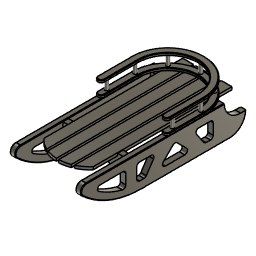
P9 (Autodesk Fusion 360 design; units mm, degrees)
Autodesk Fusion 360 part; units mm, degrees
ref_plane "WorkPlane1" through (300, 0, 0) normal (1, 0, 0) x (0, 1, 0)
sketch "Sketch1" plane through (300, 0, 0) normal (1, 0, 0) x (0, 1, 0)
  arc A0 (-924.4998, 0) -> (-300, -300) centre (-300, 500) ccw
  line L0 (-300, -300) -> (500, -300)
  line L1 (0, 0) -> (0, -300) construction
  line L2 (-924.4998, 0) -> (0, 0)
  line L3 (450, 0) -> (0, 0)
  arc A1 (500, -300) -> (650, -150) centre (500, -150) ccw
  line L4 (650, -150) -> (600, -150)
  arc A2 (450, 0) -> (600, -150) centre (600, 0) ccw
  point P0 (600, 0)
  point P1 (600, 0)
  dimension "d3" = 500
  dimension "d4" = 800
  dimension "d6" = 450
  dimension "d7" = 800
  dimension "d8" = 150
  dimension "d9" = 300
  constraint horizontal L0
  constraint tangent A0 L0
  constraint coincident L0 L1.end
  constraint vertical L1
  constraint coincident L1.start L2.end
  constraint horizontal L2
  constraint horizontal L3
  constraint tangent L0 A1
  constraint horizontal L4
  constraint tangent L4 A2
  constraint equal A1 A2
  constraint coincident P1 P0
  constraint horizontal L1.start P1
  measures "d3" distance of L0.end L1.end
  measures "d4" radius of A0
  measures "d6" distance of L3.start L1.start
  measures "d7" distance of A0.end L0.end
  measures "d8" radius of A1
  measures "d9" distance of L0 L3
extrude "Extrude1" add sketch "Sketch1" along normal mid plane 50 makes body 1
fillet "Fillet1" radius 50 1 edges at (300, -924.4998, 0) on bodies 1
mirror "Mirror1" about plane through (0, 0, 0) normal (1, 0, 0) of bodies 1 makes body 2
sketch "Sketch2" plane through (325, 0, 0) normal (1, 0, 0) x (0, 1, 0)
  arc A0 (-809.902, 0) -> (-843.8954, -86.6667) centre (-809.902, -50) ccw
  arc A1 (-843.8954, -86.6667) -> (-300, -300) centre (-300, 500) ccw
  line L0 (-300, -300) -> (500, -300)
  arc A2 (500, -300) -> (650, -150) centre (500, -150) ccw
  line L1 (650, -150) -> (600, -150)
  arc A3 (450, 0) -> (600, -150) centre (600, 0) ccw
  line L2 (450, 0) -> (-809.902, 0)
  line L3 (0, 0) -> (0, -300) construction
  line L4 (150, -225) -> (-150, -225)
  line L5 (-350, -75) -> (-350, -225)
  line L6 (-350, -225) -> (-270, -225)
  line L7 (-270, -225) -> (-170, -75)
  line L8 (-170, -75) -> (-350, -75)
  line L9 (270, -225) -> (170, -75)
  line L10 (170, -75) -> (350, -75)
  line L11 (350, -75) -> (350, -225)
  line L12 (350, -225) -> (270, -225)
  line L13 (-450, -75) -> (-760, -75)
  line L14 (-450, -75) -> (-450, -225)
  arc A4 (-760, -75) -> (-450, -225) centre (-291.5323, 497.8333) ccw
  line L15 (-150, -225) -> (0, -75)
  line L16 (150, -225) -> (0, -75)
  dimension "d17" = 300
  dimension "d18" = 75
  dimension "d19" = 80
  dimension "d20" = 180
  dimension "d23" = 350
  dimension "d24" = 740
  dimension "d25" = 75
  dimension "d26" = 310
  dimension "d27" = 450
  dimension "d28" = 75
  constraint coincident L3.start origin
  constraint coincident L0 L3.end
  constraint vertical L3
  constraint horizontal L8
  constraint collinear L4 L6
  constraint symmetric L3 L5.start L10.end
  constraint symmetric L3 L5.end L11.end
  constraint symmetric L3 L6.end L9.start
  constraint symmetric L3 L7.end L9.end
  constraint horizontal L13
  constraint perpendicular L13 L14
  constraint equal L5 L14
  constraint collinear L8 L13
  constraint coincident L3 L15.end
  constraint perpendicular L15 L16
  measures "d17" distance of L4.start L4.end
  measures "d18" distance of L0 L4
  measures "d19" distance of L5.end L6.end
  measures "d20" distance of L5.start L7.end
  measures "d23" distance of L3 L5
  measures "d24" radius of A4
  measures "d25" distance of L2 L13
  measures "d26" distance of L13.end L14
  measures "d27" distance of L3 L14
  measures "d28" distance of L2 L15.end
extrude "Extrude2" cut sketch "Sketch2" against normal blind 650 contours L4 L15 L16 | L5 L6 L7 L8 | L9 L10 L11 L12 | L13 L14 A4 bodies 1 2
fillet "Fillet2" radius 25 28 edges at (300, -450, -75) (300, -450, -225) (300, -760, -75) (300, -350, -225) (300, -270, -225) (300, -350, -75) (300, -170, -75) (300, 0, -75) (300, 150, -225) (300, -150, -225) (300, 170, -75) (300, 270, -225) (300, 350, -225) (300, 350, -75) (-300, 350, -75) (-300, 0, -75) (-300, 350, -225) (-300, 150, -225) (-300, 270, -225) (-300, -150, -225) (-300, 170, -75) (-300, -350, -75) (-300, -760, -75) (-300, -170, -75) (-300, -270, -225) (-300, -450, -225) (-300, -450, -75) (-300, -350, -225) on bodies 1 2
fillet "Fillet3" radius 5 20 edges at (325, -179.951, 0) (325, -856.4494, -31.7426) (325, -592.1187, -244.7595) (325, 100, -300) (325, 606.066, -256.066) (275, 606.066, -256.066) (275, 100, -300) (275, -592.1187, -244.7595) (275, -856.4494, -31.7426) (275, -179.951, 0) (-275, 606.066, -256.066) (-275, 100, -300) (-275, -592.1187, -244.7595) (-275, -856.4494, -31.7426) (-275, -179.951, 0) (-325, -179.951, 0) (-325, -856.4494, -31.7426) (-325, -592.1187, -244.7595) (-325, 100, -300) (-325, 606.066, -256.066) on bodies 1 2
ref_plane "WorkPlane2" through (0, -425, 0) normal (0, 1, 0) x (0, 0, 1)
sketch "Sketch3" plane through (0, -425, 0) normal (0, 1, 0) x (1, 0, 0)
  line L0 (-275, 5) -> (-225, 5)
  line L1 (-225, 5) -> (-225, 25)
  line L2 (-225, 25) -> (-2.6918, 25)
  line L3 (-275, 5) -> (-275, 155)
  line L4 (-275, 155) -> (-198.4313, 155)
  line L5 (0, 0) -> (0, 80) construction
  arc A0 (-198.4313, 155) -> (0, 80) centre (0, 380) ccw
  line L6 (225, 25) -> (2.6918, 25)
  line L7 (225, 5) -> (225, 25)
  line L8 (275, 5) -> (225, 5)
  line L9 (275, 5) -> (275, 155)
  line L10 (275, 155) -> (198.4313, 155)
  arc A1 (0, 80) -> (198.4313, 155) centre (0, 380) ccw
  line L11 (-2.6918, 25) -> (0, 25)
  line L12 (0, 25) -> (2.6918, 25)
  point P0 (-275, 5)
  point P1 (-275, 5)
  point P2 (-325, 5)
  dimension "d36" = 150
  dimension "d37" = 5
  dimension "d38" = 50
  dimension "d39" = 20
  dimension "d40" = 300
  dimension "d41" = 80
  dimension "d42" = 50
  constraint horizontal L0
  constraint perpendicular L0 L1
  constraint perpendicular L1 L2
  constraint coincident L5.start origin
  constraint vertical L5
  constraint coincident P0 L0.start
  constraint symmetric P0 L5 L8.start
  constraint symmetric L0.end L5 L7.start
  constraint symmetric L1.end L5 L6.start
  constraint symmetric L2.end L5 L6.end
  constraint symmetric L4.end L5 L10.end
  constraint symmetric L5 A0.end A1.start
  constraint symmetric L5 A0 A1
  constraint tangent A0 A1
  constraint perpendicular L0 L3
  constraint coincident P1 P0
  constraint collinear L4 L10
  constraint perpendicular L9 L10
  constraint coincident L5 L11.end
  constraint perpendicular L5 L11
  constraint perpendicular L5 L12
  measures "d36" distance of P0 L3.end
  measures "d37" vertical distance of L5.start P1
  measures "d38" distance of P0 L0.end
  measures "d39" distance of L0 L2
  measures "d40" radius of A0
  measures "d41" distance of L5.start L5.end
  measures "d42" distance of P1 P2
extrude "Extrude3" add sketch "Sketch3" along normal blind 50 separate body makes body 3
mirror "Mirror2" about plane through (0, 0, 0) normal (0, 1, 0) of bodies 3 makes body 4
sketch "Sketch4" plane through (0, 0, 0) normal (0, 0, 1) x (-1, 0, 0)
  line L0 (320, -450) -> (320, 809.902)
  line L1 (320, 809.902) -> (280, 809.902)
  line L2 (280, 809.902) -> (280, -450)
  line L3 (280, -450) -> (320, -450)
  line L4 (-127.5, 760) -> (-225, 760)
  line L5 (-275, -450.0834) -> (-275, 809.902)
  line L6 (-225, 760) -> (-225, -620)
  line L7 (0, 0) -> (-225, 0) construction
  line L8 (-127.5, 760) -> (-127.5, -620)
  line L9 (-127.5, -620) -> (-225, -620)
  line L10 (-10, 760) -> (-10, -620)
  line L11 (-10, -620) -> (-107.5, -620)
  line L12 (-107.5, 760) -> (-107.5, -620)
  line L13 (-10, 760) -> (-107.5, 760)
  line L14 (107.5, 760) -> (107.5, -620)
  line L15 (107.5, -620) -> (10, -620)
  line L16 (10, 760) -> (10, -620)
  line L17 (107.5, 760) -> (10, 760)
  line L18 (225, 760) -> (225, -620)
  line L19 (225, -620) -> (127.5, -620)
  line L20 (127.5, 760) -> (127.5, -620)
  line L21 (225, 760) -> (127.5, 760)
  dimension "d47" = 97.5
  dimension "d48" = 50
  dimension "d49" = 1380
  dimension "d50" = 620
  dimension "d54" = 117.5
  dimension "d55" = 0
  constraint horizontal L4
  constraint perpendicular L4 L6
  constraint coincident L7.start origin
  constraint coincident L6 L7.end
  constraint perpendicular L6 L7
  constraint perpendicular L4 L8
  constraint horizontal L9
  measures "d47" distance of L4.start L4.end
  measures "d48" distance of L4.end L5
  measures "d49" distance of L4.end L6.end
  measures "d50" vertical distance of L7.start L6.end
extrude "Extrude4" add sketch "Sketch4" against normal blind 25 separate body contours L4 L6 L8 L9 | L10 L11 L12 L13 | L14 L15 L16 L17 | L18 L19 L20 L21 makes body 5 at (-75, 160, 0) makes body 6 at (42.5, 160, 0) makes body 7 at (-192.5, 160, 0) makes body 8 at (160, 160, 0)
sketch "Sketch5" plane through (0, 0, 0) normal (0, 0, 1) x (1, 0, 0)
  line L0 (0, 0) -> (0, -450) construction
  arc A0 (-300, -450) -> (300, -450) centre (0, -450) ccw
  line L1 (-300, -450) -> (-300, -760)
  line L2 (300, -450) -> (300, -760)
  line L3 (-300, -760) -> (-125, -760)
  line L4 (-125, -760) -> (300, -760)
  dimension "d58" = 450
  dimension "d60" = 300
  dimension "d61" = 310
  constraint coincident L0.start origin
  constraint vertical L0
  constraint coincident L0.end A0.centre
  constraint tangent A0 L1
  constraint tangent A0 L2
  constraint vertical L1
  constraint perpendicular L1 L3
  constraint perpendicular L2 L4
  constraint collinear L3 L4
  measures "d58" distance of L0.start L0.end
  measures "d60" radius of A0
  measures "d61" distance of A0.end L2.end
extrude "Extrude5" cut sketch "Sketch5" against normal blind 25 bodies 5 6 7 8
sketch "Sketch6" plane through (0, 0, 0) normal (0, 0, 1) x (1, 0, 0)
  line L0 (0, 0) -> (0, 260) construction
  arc A0 (270, 260) -> (-270, 260) centre (0, 260) ccw
  line L1 (0, 0) -> (324.3586, 0) construction
  arc A1 (330, 260) -> (-330, 260) centre (0, 260) ccw
  line L2 (270, 260) -> (270, 0)
  line L3 (330, 260) -> (330, 0)
  line L4 (330, 0) -> (330, -50)
  line L5 (270, 0) -> (270, -50)
  arc A2 (270, -50) -> (330, -50) centre (300, -50) ccw
  line L6 (-270, 260) -> (-270, 0)
  line L7 (-270, 0) -> (-269.9822, -49.9893)
  line L8 (-330, 260) -> (-330, 0)
  line L9 (-330, 0) -> (-329.9859, -50.0085)
  arc A3 (-329.9859, -50.0085) -> (-269.9822, -49.9893) centre (-299.9841, -50) ccw
  dimension "d64" = 260
  dimension "d67" = 270
  dimension "d70" = 60
  dimension "d72" = 50
  constraint coincident L0.start L1.start
  constraint vertical L0
  constraint perpendicular L0 L1
  constraint coincident L1 L2.end
  constraint tangent A0 L2
  constraint perpendicular L1 L2
  constraint tangent A1 L3
  constraint perpendicular L1 L3
  constraint perpendicular L1 L5
  constraint tangent L5 A2
  constraint vertical L8
  constraint tangent L9 A3
  constraint tangent L7 A3
  constraint tangent A0 L6
  constraint horizontal A2.centre A3.centre
  measures "d64" distance of L0.start L0.end
  measures "d67" radius of A0
  measures "d72" vertical distance of L3.end A2.centre
extrude "Extrude6" add sketch "Sketch6" along normal blind 25 separate body makes body 9
fillet "Fillet4" radius 5 20 edges at (270, 105, 25) (300, -80, 25) (330, 105, 25) (0, 590, 25) (-330, 130, 25) (-329.9929, -25.0042, 25) (-299.9745, -80.0018, 25) (-269.9911, -24.9947, 25) (-270, 130, 25) (0, 530, 25) (-299.9745, -80.0018, 0) (-329.9929, -25.0042, 0) (-330, 130, 0) (0, 590, 0) (330, 105, 0) (300, -80, 0) (270, 105, 0) (0, 530, 0) (-270, 130, 0) (-269.9911, -24.9947, 0) on bodies 9
sketch "Sketch7" plane through (0, 0, 25) normal (0, 0, 1) x (-1, 0, 0)
  line L0 (-275, -260) -> (-275, 50)
  arc A0 (-275, 50) -> (-325, 50) centre (-300, 50) ccw
  line L1 (-325, 50) -> (-325, -260)
  arc A1 (-325, -260) -> (325, -260) centre (0, -260) ccw
  line L2 (325, -260) -> (325, -0.0007)
  line L3 (325, -0.0007) -> (324.9859, 50.0071)
  arc A2 (324.9859, 50.0071) -> (274.9822, 49.9911) centre (299.9841, 50) ccw
  line L4 (274.9822, 49.9911) -> (275, 0.0009)
  line L5 (275, 0.0009) -> (275, -260)
  arc A3 (-275, -260) -> (275, -260) centre (0, -260) ccw
  line L6 (0, 0) -> (300, 0.0847) construction
  circle A4 centre (300, 0.0847) radius 15
  line L7 (0, 0) -> (-300, 0) construction
  circle A5 centre (-300, 0) radius 15
  line L8 (300, 0.0847) -> (300.0734, -259.9153) construction
  circle A6 centre (300.0734, -259.9153) radius 15
  circle A7 centre (212.2438, -472.124) radius 15
  circle A8 centre (0.0847, -560.0734) radius 15
  circle A9 centre (-212.124, -472.2438) radius 15
  circle A10 centre (-300.0734, -260.0847) radius 15
  dimension "d77" = 300
  dimension "d78" = 30
  dimension "d79" = 300
  dimension "d80" = 30
  dimension "d81" = 260
  dimension "d82" = 30
  dimension "d84" = -180
  constraint coincident L6.start L7.start
  constraint perpendicular L3 L6
  constraint coincident L6.end A4.centre
  constraint perpendicular L0 L7
  constraint coincident L7.end A5.centre
  constraint perpendicular L6 L8
  constraint coincident L8.end A6.centre
  measures "d77" distance of L6.start L6.end
  measures "d78" diameter of A4
  measures "d79" distance of L6.start L7.end
  measures "d80" diameter of A5
  measures "d81" distance of L6.end L8.end
  measures "d82" diameter of A6
extrude "Extrude7" add sketch "Sketch7" along normal blind 105 separate body contours A4 | A5 | A6 | A7 | A8 | A9 | A10 makes body 10 at (197.5879, 468.5425, 95) makes body 11 at (-314.9254, 1.4088, 95) makes body 12 at (-10.01, 548.8267, 95) makes body 13 at (314.9988, 261.5782, 95) makes body 14 at (-285.1479, 261.4088, 95) makes body 15 at (-226.78, 468.4227, 95) makes body 16 at (285.0745, 1.4935, 95)
pattern_linear "R-Pattern1" count 2 spacing 120 along (0, 0, 1) of bodies 9 makes body 17
